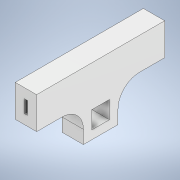
# Autodesk Inventor part: fuselage_wing_interface_2
Saved by Autodesk Inventor 2021 (Build 250183000, 183)
## iProperties
Created: 2020-11-15
Part Number: fuselage_wing_interface_2
Material: ABS Plastic
Document SubType Name: Modeling
Designer: Paco
Density: 1.06 g/cm^3
Appearance: Smooth - White
Mass: 2.34604 g
Surface Area: 16.1332 cm^2
Volume: 2.21324 cm^3
Author: Paco
Autodesk Inventor part; units mm, degrees
ref_plane "YZ Plane" through (0, 0, 0) normal (1, 0, 0) x (0, 1, 0)
ref_plane "XZ Plane" through (0, 0, 0) normal (0, 1, 0) x (-1, 0, 0)
ref_plane "XY Plane" through (0, 0, 0) normal (0, 0, 1) x (1, 0, 0)
sketch "Sketch1" plane through (0, 0, 0) normal (1, 0, 0) x (0, 1, 0)
  line L0 (4.05, 4.05) -> (-4.05, 4.05)
  line L1 (-4.05, 4.05) -> (-4.05, -4.05)
  line L2 (-4.05, -4.05) -> (4.05, -4.05)
  line L3 (4.05, -4.05) -> (4.05, 4.05)
  line L4 (11.55, 15) -> (4.05, 15)
  line L5 (4.05, 15) -> (4.05, -15)
  line L6 (4.05, -15) -> (11.55, -15)
  line L7 (11.55, -15) -> (11.55, 15)
  line L8 (4.05, 4.05) -> (-4.05, -4.05) construction
  line L9 (4.05, -4.05) -> (-4.05, 4.05) construction
  line L10 (2.05, 2.05) -> (-2.05, 2.05)
  line L11 (-2.05, 2.05) -> (-2.05, -2.05)
  line L12 (-2.05, -2.05) -> (2.05, -2.05)
  line L13 (2.05, -2.05) -> (2.05, 2.05)
  line L14 (2.05, 2.05) -> (-2.05, -2.05) construction
  line L15 (-2.05, 2.05) -> (2.05, -2.05) construction
  point P0 (4.05, 4.05)
  point P1 (0, 0)
  point P2 (0, 0)
  point P3 (0, 0)
  dimension "d0" = 8.1
  dimension "d3" = 8.1
  dimension "d22" = 10.95
  dimension "d24" = 30
  dimension "d25" = 7.5
  dimension "d55" = 10.95
  dimension "d65" = 4.1
  dimension "d66" = 4.1
  constraints: 32 end point, 6 parallel, 4 midpoint, 4 perpendicular, 3 horizontal, 1 coincident, 1 collinear, 1 point on line, 1 other
  measures "d0" distance of L2.end L0.start
  measures "d3" distance of L1.end L2.end
  measures "d22" distance between parallel lines of L0 L4
  measures "d24" distance of L6.end L4.start
  measures "d25" distance of L5.end L6.end
  measures "d55" distance between parallel lines of L2 L6
  measures "d65" distance of L12.end L10.start
  measures "d66" distance of L11.end L12.end
extrude "Extrusion1" add sketch "Sketch1" along normal blind 5
sketch "Sketch5" plane through (0, 4.05, 15) normal (0, 0, 1) x (1, 0, 0)
  line L0 (2.15, 5.25) -> (2.85, 5.25)
  line L1 (2.85, 5.25) -> (2.85, 2.25)
  line L2 (2.85, 2.25) -> (2.15, 2.25)
  line L3 (2.15, 2.25) -> (2.15, 5.25)
  line L4 (0, 0) -> (5, 0) projected
  line L5 (0, 7.5) -> (0, 0) projected
  point P0 (0, -4.05)
  dimension "d86" = 3
  dimension "d87" = 0.7
  dimension "d88" = 2.25
  dimension "d89" = 2.15
  constraints: 8 end point, 2 parallel, 1 horizontal, 1 perpendicular
  measures "d86" distance of L0.end L1.end
  measures "d87" distance of L1.end L2.end
  measures "d88" distance between parallel lines of L4 L2
  measures "d89" distance between parallel lines of L5 L3
extrude "Extrusion4" cut sketch "Sketch5" against normal through all
fillet "Fillet3" radius 5 2 edges at (2.5, 4.05, 4.05) (2.5, 4.05, -4.05)
equation "\"d3\" = d0"
equation "\"d22\" = d55"
body "Solid1"
